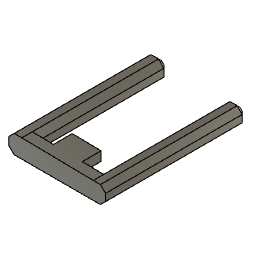
LTS_Pin_v0.1 (Autodesk Fusion 360 design; units mm, degrees)
Autodesk Fusion 360 part; units mm, degrees
note: some values were not read from the file. Set by a fixed rule: which sketch regions a step uses.
sketch "Sketch1" plane through (0, 0, 0) normal (0, 1, 0) x (1, 0, 0)
  line L0 (1.4782, -0.8659) -> (0.6123, 0)
  line L1 (-1.4782, -2.0905) -> (-0.6123, -2.9564)
  circle A0 centre (0, -1.4782) radius 1.6 construction
  line L2 (-0.6123, 0) -> (-1.4782, -0.8659)
  line L3 (0.6123, -2.9564) -> (1.4782, -2.0905)
  line L4 (-1.4782, -0.8659) -> (-1.4782, -2.0905)
  line L5 (0.6123, 0) -> (-0.6123, 0)
  line L6 (-0.6123, -2.9564) -> (0.6123, -2.9564)
  line L7 (1.4782, -2.0905) -> (1.4782, -0.8659)
  line L8 (8.6194, -1.353) -> (7.2664, 0)
  line L9 (4, -3.2664) -> (5.353, -4.6194)
  circle A1 centre (6.3097, -2.3097) radius 2.5 construction
  line L10 (5.353, 0) -> (4, -1.353)
  line L11 (7.2664, -4.6194) -> (8.6194, -3.2664)
  line L12 (4, -1.353) -> (4, -3.2664)
  line L13 (7.2664, 0) -> (5.353, 0)
  line L14 (5.353, -4.6194) -> (7.2664, -4.6194)
  line L15 (8.6194, -3.2664) -> (8.6194, -1.353)
  line L16 (0.6123, 0) -> (5.353, 0) construction
  line L17 (13.1934, -2.7716) -> (14.0052, -1.9598)
  line L18 (13.1934, 0) -> (12.0454, 0)
  line L19 (14.0052, -0.8118) -> (13.1934, 0)
  line L20 (14.0052, -1.9598) -> (14.0052, -0.8118)
  line L21 (11.2336, -0.8118) -> (11.2336, -1.9598)
  line L22 (11.2336, -1.9598) -> (12.0454, -2.7716)
  line L23 (12.0454, 0) -> (11.2336, -0.8118)
  circle A2 centre (12.6194, -1.3858) radius 1.5 construction
  line L24 (7.2664, 0) -> (12.0454, 0) construction
  line L25 (12.0454, -2.7716) -> (13.1934, -2.7716)
  line L26 (0.6123, -2.9564) -> (12.0454, -2.7716)
  point P0 (0, -1.4782)
  point P1 (6.3097, -2.3097)
  point P2 (6.3097, 0)
  point P3 (12.6194, 0)
  point P4 (12.6194, -1.3858)
  dimension "d3" = 3.2
  dimension "d4" = 5
  dimension "d11" = 4
  dimension "d12" = 3
  dimension "d13" = 4
  constraint midpoint origin L5
  constraint horizontal L5
  constraint coincident P0 A0.centre
  constraint coincident L0.end A0
  constraint midpoint P2 L13
  constraint horizontal L13
  constraint coincident P1 A1.centre
  constraint coincident L8.end A1
  constraint horizontal L16
  constraint midpoint P3 L18
  constraint horizontal L18
  constraint coincident P4 A2.centre
  constraint coincident L18.start A2
  constraint horizontal L24
  constraint coincident L8.end L13.start
  measures "d3" diameter of A0
  measures "d4" diameter of A1
  measures "d11" distance of P0 L12
  measures "d12" diameter of A2
  measures "d13" distance of L15 P4
extrude "Extrude1" add sketch "Sketch1" along normal blind 18 contours L0 L1 L2 L3 L4 L5 L6 L7 | L17 L18 L19 L20 L21 L22 L23 L25 makes body 1 at (-1.1896, 6, 2.3791) makes body 2 at (13.464, 12, 2.501)
sketch "Sketch2" plane through (0, 0, 0) normal (0, 1, 0) x (1, 0, 0)
extrude "Extrude3" add sketch "Sketch1" against normal blind 3 contours L0 L1 L2 L3 L4 L5 L6 L7 | L8 L10 L12 L13 L15 L26 | L17 L18 L19 L20 L21 L22 L23 L25 bodies 1 2 makes body 3
sketch "Sketch3" plane through (0, -3, 0) normal (0, -1, 0) x (1, 0, 0)
  line L0 (1.4782, 0.8659) -> (1.4782, 2.0905)
  line L1 (1.4782, 2.0905) -> (0.6123, 2.9564)
  line L2 (0.6123, 2.9564) -> (-0.6123, 2.9564)
  line L3 (-0.6123, 2.9564) -> (-1.4782, 2.0905)
  line L4 (-1.4782, 2.0905) -> (-1.4782, 0.8659)
  line L5 (-1.4782, 0.8659) -> (-0.6123, 0)
  line L6 (-0.6123, 0) -> (0.6123, 0)
  line L7 (0.6123, 0) -> (1.4782, 0.8659)
  line L8 (8.6194, 1.353) -> (8.6194, 2.827)
  line L9 (4, 2.9017) -> (4, 1.353)
  line L10 (4, 1.353) -> (5.353, 0)
  line L11 (5.353, 0) -> (7.2664, 0)
  line L12 (7.2664, 0) -> (8.6194, 1.353)
  line L13 (13.1934, 2.7716) -> (14.0052, 1.9598)
  line L14 (13.1934, 2.7716) -> (12.0454, 2.7716)
  line L15 (12.0454, 2.7716) -> (11.2336, 1.9598)
  line L16 (11.2336, 1.9598) -> (11.2336, 0.8118)
  line L17 (11.2336, 0.8118) -> (12.0454, 0)
  line L18 (12.0454, 0) -> (13.1934, 0)
  line L19 (13.1934, 0) -> (14.0052, 0.8118)
  line L20 (14.0052, 0.8118) -> (14.0052, 1.9598)
  line L21 (14.0052, 1.9598) -> (13.1934, 2.7716)
  line L22 (0.6123, 0) -> (5.353, 0)
  line L23 (7.2664, 0) -> (12.0454, 0)
  line L24 (8.6194, 2.827) -> (4, 2.9017)
  line L25 (12.0454, 2.7716) -> (0.6123, 2.9564)
  constraint coincident L6.end L7.start
  constraint coincident L10.end L11.start
  constraint coincident L11.end L12.start
  constraint coincident L17.end L18.start
  constraint coincident L14.end L15.start
  constraint coincident L1.end L2.start
extrude "Extrude4" add sketch "Sketch3" along normal blind 1.67 bodies 1 2 3
chamfer "Chamfer1" distance 0.8 angle 45 16 edges at (0, 18, 2.9564) (1.0453, 18, 2.5235) (1.4782, 18, 1.4782) (-1.0453, 18, 2.5235) (-1.4782, 18, 1.4782) (11.2336, 18, 1.3858) (11.6395, 18, 2.3657) (12.6194, 18, 2.7716) (13.5993, 18, 2.3657) (14.0052, 18, 1.3858) (12.6194, 18, 0) (13.5993, 18, 0.4059) (11.6395, 18, 0.4059) (1.0453, 18, 0.433) (0, 18, 0) (-1.0453, 18, 0.433) on bodies 1 2
sketch "Sketch4" plane through (14.0052, 0, 0) normal (1, 0, 0) x (0, 1, 0)
  line L0 (17.2, 0.8118) -> (17.2, 1.9598)
  line L1 (17.2, 1.9598) -> (-4.67, 1.9598)
  line L2 (-4.67, 1.9598) -> (-4.67, 0.8118)
  line L3 (-4.67, 0.8118) -> (17.2, 0.8118)
  line L4 (-3.4663, 1.9598) -> (-1.7963, 1.9598)
  line L5 (-1.7963, 1.9598) -> (-1.7963, 0.8118)
  line L6 (-1.7963, 0.8118) -> (-3.4663, 0.8118)
  line L7 (-3.4663, 0.8118) -> (-3.4663, 1.9598)
  dimension "d19" = 1.67
  constraint horizontal L4
  constraint vertical L5
  constraint horizontal L6
  constraint vertical L7
  constraint coincident L3 L5.end
  constraint coincident L1 L4.start
  measures "d19" distance of L5 L7
sketch "Label" plane through (0, -4.67, 0) normal (0, -1, 0) x (1, 0, 0)
  line L0 (-0.6123, 0) -> (13.1934, 0)
  line L1 (13.1934, 0) -> (14.0052, 0.8118)
  line L2 (14.0052, 0.8118) -> (14.0052, 1.9598)
  line L3 (14.0052, 1.9598) -> (13.1934, 2.7716)
  line L4 (13.1934, 2.7716) -> (12.0454, 2.7716)
  line L5 (12.0454, 2.7716) -> (0.6123, 2.9564)
  line L6 (0.6123, 2.9564) -> (-0.6123, 2.9564)
  line L7 (-0.6123, 2.9564) -> (-1.4782, 2.0905)
  line L8 (-1.4782, 2.0905) -> (-1.4782, 0.8659)
  line L9 (-1.4782, 0.8659) -> (-0.6123, 0)
  line L10 (0.835, 1.2924) -> (-0.835, 1.2924)
  line L11 (-0.835, 1.2924) -> (-0.835, 1.664)
  line L12 (-0.835, 1.664) -> (0.835, 1.664)
  line L13 (0.835, 1.664) -> (0.835, 1.2924)
  line L14 (0.835, 1.2924) -> (-0.835, 1.664) construction
  line L15 (-0.835, 1.2924) -> (0.835, 1.664) construction
  line L16 (13.4544, 1.2) -> (11.7844, 1.2)
  line L17 (11.7844, 1.2) -> (11.7844, 1.5716)
  line L18 (11.7844, 1.5716) -> (13.4544, 1.5716)
  line L19 (13.4544, 1.5716) -> (13.4544, 1.2)
  line L20 (13.4544, 1.2) -> (11.7844, 1.5716) construction
  line L21 (11.7844, 1.2) -> (13.4544, 1.5716) construction
  line L22 (13.1934, 0) -> (12.0454, 0)
  line L23 (0.1858, 0.6432) -> (-0.1858, 0.6432)
  line L24 (-0.1858, 0.6432) -> (-0.1858, 2.3132)
  line L25 (-0.1858, 2.3132) -> (0.1858, 2.3132)
  line L26 (0.1858, 2.3132) -> (0.1858, 0.6432)
  line L27 (0.1858, 0.6432) -> (-0.1858, 2.3132) construction
  line L28 (-0.1858, 0.6432) -> (0.1858, 2.3132) construction
  point P0 (12.6194, 1.3858)
  point P1 (0, 1.4782)
  point P2 (0, 1.4782)
  point P3 (12.6194, 1.3858)
  point P4 (0, 1.4782)
  dimension "d20" = 1.67
  dimension "d21" = 1.2
  dimension "d22" = 1.67
  constraint horizontal L10
  constraint perpendicular L10 L11
  constraint parallel L10 L12
  constraint parallel L11 L13
  constraint coincident L14 P4
  constraint coincident L15 P4
  constraint coincident P4 P2
  constraint horizontal L16
  constraint perpendicular L16 L17
  constraint parallel L16 L18
  constraint parallel L17 L19
  constraint coincident L20 P3
  constraint coincident L21 P3
  constraint coincident P3 P0
  constraint horizontal L23
  constraint perpendicular L23 L24
  constraint parallel L23 L25
  constraint parallel L24 L26
  constraint coincident L27 P4
  constraint coincident L28 P4
  constraint equal L13 L25
  constraint equal L12 L26
  constraint equal L13 L17
  measures "d20" distance of L17 L19
  measures "d21" distance of L16 L22
  measures "d22" distance of L11 L13
extrude "Extrude5" [rolled back] along distance -0.7 taper angle -45
extrude "Extrude6" [rolled back] along distance -1.4 taper angle -45
named bodies: "Pin"
